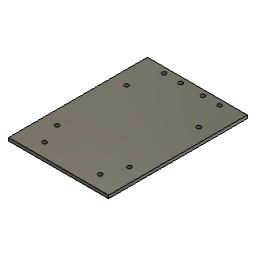
Top (Autodesk Fusion 360 design; units mm, degrees)
Autodesk Fusion 360 part; units mm, degrees
sketch "Sketch1" plane through (0, 0, 0) normal (0, 1, 0) x (1, 0, 0)
  line L0 (0, 0) -> (91.44, 0)
  line L1 (91.44, 0) -> (91.44, 127)
  line L2 (91.44, 127) -> (0, 127)
  line L3 (0, 127) -> (0, 0)
  circle A0 centre (71.12, 121.92) radius 1.905
  circle A1 centre (12.7, 31.75) radius 1.905
  circle A2 centre (78.74, 95.25) radius 1.905
  circle A3 centre (78.74, 31.75) radius 1.905
  circle A4 centre (20.32, 121.92) radius 1.905
  circle A5 centre (71.12, 12.7) radius 1.905
  circle A6 centre (35.56, 121.92) radius 1.905
  circle A7 centre (20.32, 12.7) radius 1.905
  circle A8 centre (55.88, 121.92) radius 1.905
  circle A9 centre (12.7, 95.25) radius 1.905
  circle A10 centre (45.72, 12.7) radius 1.905
  circle A11 centre (12.7, 82.55) radius 1.905
  circle A12 centre (78.74, 82.55) radius 1.905
  circle A13 centre (45.72, 38.1) radius 9.525
  dimension "d1" = 91.44
  dimension "d54" = 3.81
  dimension "d57" = 3.81
  dimension "d60" = 3.81
  dimension "d61" = 19.05
  constraint horizontal L0
  constraint vertical L1
  constraint horizontal L2
  constraint vertical L3
  constraint coincident L0.start L3.end
  measures "d1" distance of L0.start L0.end
  measures "d54" diameter of A10
  measures "d57" diameter of A11
  measures "d60" diameter of A12
  measures "d61" diameter of A13
extrude "Extrude4" add sketch "Sketch1" along normal blind 2.794 contours L0 L1 L2 L3 | A10 | A11 | A12 | A13
